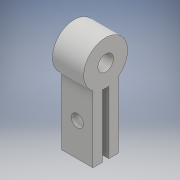
# Autodesk Inventor part: servo attachment
Saved by Autodesk Inventor 2017 (Build 210142000, 142)
## iProperties
Created: 2017-04-28
Part Number: servo attachment
Material: Generic
Document SubType Name: Modeling
Designer: s4321966
Density: 1 g/cm^3
Appearance: Default
Author: s4321966
Autodesk Inventor part; units mm, degrees
ref_plane "YZ Plane" through (0, 0, 0) normal (1, 0, 0) x (0, 1, 0)
ref_plane "XZ Plane" through (0, 0, 0) normal (0, 1, 0) x (-1, 0, 0)
ref_plane "XY Plane" through (0, 0, 0) normal (0, 0, 1) x (1, 0, 0)
sketch "Sketch1" plane through (0, 0, 0) normal (1, 0, 0) x (0, 1, 0)
  circle A0 centre (0, 0) radius 3.5
  circle A1 centre (0, 0) radius 1.25
  line L0 (0, -3.5) -> (0.5, -3.5)
  line L1 (0.5, -3.5) -> (0.5, -13.5)
  line L2 (0.5, -13.5) -> (0, -13.5)
  line L3 (0, -13.5) -> (0, -3.5)
  line L4 (0.5, -13.5) -> (2.0279, -13.5)
  line L5 (2.0279, -13.5) -> (2.0279, -5.25)
  line L6 (2.0279, -5.25) -> (0.5, -5.25)
  line L7 (0.5, -5.25) -> (0.5, -13.5)
  line L8 (0, -3.5) -> (-0.5, -3.5)
  line L9 (-0.5, -3.5) -> (-0.5, -13.5)
  line L10 (-0.5, -13.5) -> (0, -13.5)
  line L11 (-0.5, -13.5) -> (-2.0279, -13.5)
  line L12 (-2.0279, -13.5) -> (-2.0279, -5.25)
  line L13 (-2.0279, -5.25) -> (-0.5, -5.25)
  line L14 (-0.5, -5.25) -> (-0.5, -13.5)
  line L15 (-0.5, -13.5) -> (-2.0279, -13.5)
  line L16 (-2.0279, -13.5) -> (-2.0279, -2.6024)
  line L17 (-2.0279, -2.6024) -> (-0.5, -2.6024)
  line L18 (-0.5, -2.6024) -> (-0.5, -13.5)
  line L19 (2.0279, -13.5) -> (0.5, -13.5)
  line L20 (0.5, -13.5) -> (0.5, -2.6024)
  line L21 (0.5, -2.6024) -> (2.0279, -2.6024)
  line L22 (2.0279, -2.6024) -> (2.0279, -13.5)
  dimension "d0" = 7
  dimension "d1" = 2.5
  dimension "d2" = 0.5
  dimension "d3" = 10
  constraints: 46 end point, 8 parallel, 5 symmetric about line, 4 coincident, 4 horizontal, 4 perpendicular, 3 point on line, 1 centre point, 1 vertical alignment, 2 other
  measures "d1" diameter of A1
  measures "d2" distance of L1.end L2.end
  measures "d3" distance of L0.end L1.end
extrude "Extrusion1" add sketch "Sketch1" along normal blind 5 contours A0 L22 L21 L20 L18 L17 L16 | L16 L17 L18 A0 | A0 L18 L9 L13 L16 | L22 L6 L1 L20 A0 | A0 L20 L21 L22 | L13 L9 L11 L12 | L5 L4 L1 L6
sketch "Sketch3" plane through (0, 2.0279, -2.8527) normal (0, 1, 0) x (1, 0, 0)
  line L0 (0, 0) -> (5.024, 10.7024)
  circle A0 centre (2.512, 5.3512) radius 0.9732
  point P0 (0, -2.8527)
  constraints: 2 end point, 1 centre point, 1 midpoint
extrude "Extrusion3" cut sketch "Sketch3" against normal blind 10
body "Solid1"
